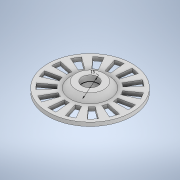
# Autodesk Inventor part: rotary encoder
Saved by Autodesk Inventor 2020.3 (Build 243373000, 373)
## iProperties
Created: 2020-08-18
Part Number: rotary encoder
Material: Generic
Document SubType Name: Modeling
Designer: joesp
Density: 1 g/cm^3
Appearance: Default
Author: joesp
Autodesk Inventor part; units mm, degrees
ref_plane "YZ Plane" through (0, 0, 0) normal (1, 0, 0) x (0, 1, 0)
ref_plane "XZ Plane" through (0, 0, 0) normal (0, 1, 0) x (-1, 0, 0)
ref_plane "XY Plane" through (0, 0, 0) normal (0, 0, 1) x (1, 0, 0)
sketch "Sketch1" plane through (0, 0, 0) normal (0, 1, 0) x (-1, 0, 0)
  circle A0 centre (0, 0) radius 12.5
  circle A1 centre (0, 0) radius 22.5
  line L0 (12.5, 0) -> (22.5, 0)
  line L1 (12.2268, 2.5989) -> (22.0083, 4.678)
  line L2 (11.4193, 5.0842) -> (20.5548, 9.1516)
  line L3 (10.1127, 7.3473) -> (18.2029, 13.2252)
  line L4 (8.3641, 9.2893) -> (15.0554, 16.7208)
  line L5 (6.25, 10.8253) -> (11.25, 19.4856)
  line L6 (3.8627, 11.8882) -> (6.9529, 21.3988)
  line L7 (1.3066, 12.4315) -> (2.3519, 22.3767)
  line L8 (-1.3066, 12.4315) -> (-2.3519, 22.3767)
  line L9 (-3.8627, 11.8882) -> (-6.9529, 21.3988)
  line L10 (-6.25, 10.8253) -> (-11.25, 19.4856)
  line L11 (-8.3641, 9.2893) -> (-15.0554, 16.7208)
  line L12 (-10.1127, 7.3473) -> (-18.2029, 13.2252)
  line L13 (-11.4193, 5.0842) -> (-20.5548, 9.1516)
  line L14 (-12.2268, 2.5989) -> (-22.0083, 4.678)
  line L15 (-12.5, 0) -> (-22.5, 0)
  line L16 (-12.2268, -2.5989) -> (-22.0083, -4.678)
  line L17 (-11.4193, -5.0842) -> (-20.5548, -9.1516)
  line L18 (-10.1127, -7.3473) -> (-18.2029, -13.2252)
  line L19 (-8.3641, -9.2893) -> (-15.0554, -16.7208)
  line L20 (-6.25, -10.8253) -> (-11.25, -19.4856)
  line L21 (-3.8627, -11.8882) -> (-6.9529, -21.3988)
  line L22 (-1.3066, -12.4315) -> (-2.3519, -22.3767)
  line L23 (1.3066, -12.4315) -> (2.3519, -22.3767)
  line L24 (3.8627, -11.8882) -> (6.9529, -21.3988)
  line L25 (6.25, -10.8253) -> (11.25, -19.4856)
  line L26 (8.3641, -9.2893) -> (15.0554, -16.7208)
  line L27 (10.1127, -7.3473) -> (18.2029, -13.2252)
  line L28 (11.4193, -5.0842) -> (20.5548, -9.1516)
  line L29 (12.2268, -2.5989) -> (22.0083, -4.678)
  circle A2 centre (0, 0) radius 4.25
  circle A3 centre (0, 0) radius 20.5
  point P0 (18.7277, 8.3381)
  point P1 (20.052, 4.2622)
  point P2 (20.5, 0)
  point P3 (20.052, -4.2622)
  point P4 (18.7277, -8.3381)
  point P5 (16.5848, -12.0496)
  point P6 (13.7172, -15.2345)
  point P7 (10.25, -17.7535)
  point P8 (6.3348, -19.4967)
  point P9 (2.1428, -20.3877)
  point P10 (-2.1428, -20.3877)
  point P11 (-6.3348, -19.4967)
  point P12 (-10.25, -17.7535)
  point P13 (-13.7172, -15.2345)
  point P14 (-16.5848, -12.0496)
  point P15 (-18.7277, -8.3381)
  point P16 (-20.052, -4.2622)
  point P17 (-20.5, 0)
  point P18 (-20.052, 4.2622)
  point P19 (-18.7277, 8.3381)
  point P20 (-16.5848, 12.0496)
  point P21 (-13.7172, 15.2345)
  point P22 (-10.25, 17.7535)
  point P23 (-6.3348, 19.4967)
  point P24 (-2.1428, 20.3877)
  point P25 (2.1428, 20.3877)
  point P26 (6.3348, 19.4967)
  point P27 (10.25, 17.7535)
  point P28 (13.7172, 15.2345)
  point P29 (16.5848, 12.0496)
  dimension "d0" = 45
  dimension "d1" = 10
  dimension "d17" = 2
  dimension "d6" = 360
  dimension "d11" = 8.5
  constraints: 60 end point, 5 coincident, 1 centre point, 1 horizontal, 1 horizontal alignment, 99 other
  measures "d11" diameter of A2
extrude "Extrusion1" add sketch "Sketch1" along normal blind 2 contours A0 | A0 L1 A3 L0 | L29 A3 L28 A0 | A3 L1 A1 L0 | L0 A1 L29 A3 | A0 L3 A3 L2 | A3 L2 A1 L1 | L29 A1 L28 A3 | A3 L3 A1 L2 | L27 A3 L26 A0 | L28 A1 L27 A3 | A0 L5 A3 L4 | A3 L4 A1 L3 | L27 A1 L26 A3 | A3 L5 A1 L4 | L25 A3 L24 A0 | L26 A1 L25 A3 | A0 L7 A3 L6 | A3 L6 A1 L5 | L25 A1 L24 A3 | A3 L7 A1 L6 | L23 A3 L22 A0 | L24 A1 L23 A3 | A0 L9 A3 L8 | A3 L8 A1 L7 | L23 A1 L22 A3 | A3 L9 A1 L8 | L21 A3 L20 A0 | L22 A1 L21 A3 | A0 L11 A3 L10 | A3 L10 A1 L9 | L21 A1 L20 A3 | A3 L11 A1 L10 | L19 A3 L18 A0 | L20 A1 L19 A3 | A0 L13 A3 L12 | A3 L12 A1 L11 | L19 A1 L18 A3 | A3 L13 A1 L12 | L17 A3 L16 A0 | L18 A1 L17 A3 | A0 L15 A3 L14 | A3 L14 A1 L13 | L17 A1 L16 A3 | A3 L15 A1 L14 | L16 A1 L15 A3
sketch "Sketch3" plane through (0, 2, 0) normal (0, 1, 0) x (1, 0, 0)
  circle A0 centre (0, 0) radius 4.25
  circle A1 centre (0, 0) radius 7.5
  circle A2 centre (0, 0) radius 4.25 projected
  dimension "d19" = 15
  constraints: 2 centre point, 2 coincident, 1 concentric
  measures "d19" diameter of A1
extrude "Extrusion3" add sketch "Sketch3" along normal blind 3 and the other way blind 5
chamfer "Chamfer2" distance 3 angle 45 2 edges at (-7.5, 2, 0) (-7.5, 0, 0)
body "Solid1"
